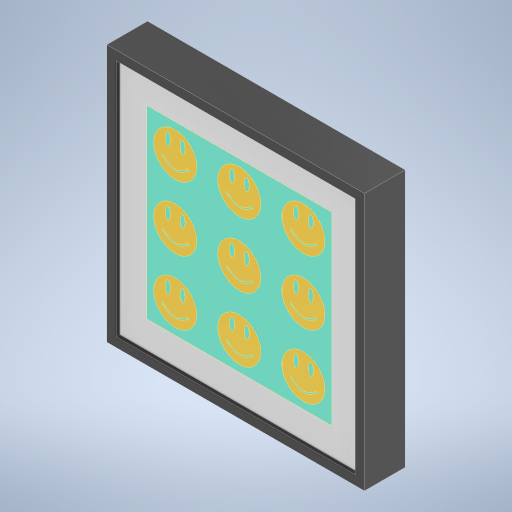
# Autodesk Inventor part: picture-frame-square
Saved by Autodesk Inventor 2023 (Build 270158030, 158C)
## iProperties
Created: 2023-12-24
Part Number: picture-frame-square
Material: Generic
Document SubType Name: Modeling
Designer: Imogen Heard
Density: 1 g/cm^3
Appearance: Glossy - Gold
Author: Imogen Heard
Autodesk Inventor part; units mm, degrees
ref_plane "YZ Plane" through (0, 0, 0) normal (1, 0, 0) x (0, 1, 0)
ref_plane "XZ Plane" through (0, 0, 0) normal (0, 1, 0) x (-1, 0, 0)
ref_plane "XY Plane" through (0, 0, 0) normal (0, 0, 1) x (1, 0, 0)
sketch "Sketch1" plane through (0, 0, 0) normal (0, 0, 1) x (1, 0, 0)
  line L0 (0, 200) -> (200, 200)
  line L1 (200, 200) -> (200, 0)
  line L2 (200, 0) -> (0, 0)
  line L3 (0, 0) -> (0, 200)
  dimension "d0" = 200
  dimension "d1" = 200
  constraints: 8 end point, 2 parallel, 1 coincident, 1 horizontal, 1 perpendicular
  measures "d0" distance between parallel lines of L1 L3
  measures "d1" distance between parallel lines of L2 L0
extrude "Extrusion1" add sketch "Sketch1" along normal blind 0.01
sketch "Sketch2" plane through (0, 0, 0.01) normal (0, 0, 1) x (1, 0, 0)
  line L0 (25, 175) -> (175, 175)
  line L1 (175, 175) -> (175, 25)
  line L2 (175, 25) -> (25, 25)
  line L3 (25, 25) -> (25, 175)
  line L4 (0, 200) -> (0, 0) projected
  line L5 (200, 200) -> (0, 200) projected
  line L6 (200, 0) -> (200, 200) projected
  line L7 (0, 0) -> (200, 0) projected
  dimension "d4" = 25
  dimension "d5" = 25
  dimension "d6" = 25
  dimension "d7" = 25
  constraints: 8 end point, 2 parallel, 1 horizontal, 1 perpendicular
  measures "d4" distance between parallel lines of L4 L3
  measures "d5" distance between parallel lines of L5 L0
  measures "d6" distance between parallel lines of L6 L1
  measures "d7" distance between parallel lines of L7 L2
extrude "Extrusion2" add sketch "Sketch2" along normal blind 0.02 contours L0 L1 L2 L3
sketch "Sketch3" plane through (0, 0, 0.03) normal (0, 0, 1) x (1, 0, 0)
  circle A0 centre (48, 152) radius 17.5
  line L0 (175, 175) -> (25, 175) projected
  line L1 (25, 175) -> (25, 25) projected
  ellipse E0 centre (42, 160) end of major axis (42, 155) minor radius 2
  ellipse E1 centre (54, 160) end of major axis (54, 155) minor radius 2
  line L2 (38.6458, 146.4746) -> (47.8499, 137.8273) construction
  line L3 (47.8499, 137.8273) -> (57.4024, 146.0108) construction
  spline S0 degree 2 poles (38.6458, 146.4746) (47.8499, 137.8273) (57.4024, 146.0108) knots 1 1 1 2 2 2
  ellipse E2 centre (58.0984, 145.8999) end of major axis (58.7934, 145.0887) minor radius 0.5281 (58.0325, 145.2429) -> (57.4024, 146.0108) ccw
  ellipse E3 centre (37.9912, 146.4065) end of major axis (38.6402, 147.2549) minor radius 0.5281 (38.6458, 146.4746) -> (38.0218, 145.6984) ccw
  ellipse E4 centre (89.9912, 146.4065) end of major axis (90.6402, 147.2549) minor radius 0.5281 (90.6458, 146.4746) -> (90.0218, 145.6984) ccw
  ellipse E5 centre (110.0984, 145.8999) end of major axis (110.7934, 145.0887) minor radius 0.5281 (110.0325, 145.2429) -> (109.4024, 146.0108) ccw
  spline S1 degree 2 poles (90.6458, 146.4746) (99.8499, 137.8273) (109.4024, 146.0108) knots 1 1 1 2 2 2
  line L4 (90.6458, 146.4746) -> (99.8499, 137.8273) construction
  line L5 (99.8499, 137.8273) -> (109.4024, 146.0108) construction
  circle A1 centre (100, 152) radius 17.5
  ellipse E6 centre (94, 160) end of major axis (94, 155) minor radius 2
  ellipse E7 centre (106, 160) end of major axis (106, 155) minor radius 2
  ellipse E8 centre (141.9912, 146.4065) end of major axis (142.6402, 147.2549) minor radius 0.5281 (142.6458, 146.4746) -> (142.0218, 145.6984) ccw
  ellipse E9 centre (162.0984, 145.8999) end of major axis (162.7934, 145.0887) minor radius 0.5281 (162.0325, 145.2429) -> (161.4024, 146.0108) ccw
  spline S2 degree 2 poles (142.6458, 146.4746) (151.8499, 137.8273) (161.4024, 146.0108) knots 1 1 1 2 2 2
  line L6 (142.6458, 146.4746) -> (151.8499, 137.8273) construction
  line L7 (151.8499, 137.8273) -> (161.4024, 146.0108) construction
  circle A2 centre (152, 152) radius 17.5
  ellipse E10 centre (146, 160) end of major axis (146, 155) minor radius 2
  ellipse E11 centre (158, 160) end of major axis (158, 155) minor radius 2
  ellipse E12 centre (37.9912, 94.4065) end of major axis (38.6402, 95.2549) minor radius 0.5281 (38.6458, 94.4746) -> (38.0218, 93.6984) ccw
  ellipse E13 centre (58.0984, 93.8999) end of major axis (58.7934, 93.0887) minor radius 0.5281 (58.0325, 93.2429) -> (57.4024, 94.0108) ccw
  spline S3 degree 2 poles (38.6458, 94.4746) (47.8499, 85.8273) (57.4024, 94.0108) knots 1 1 1 2 2 2
  line L8 (38.6458, 94.4746) -> (47.8499, 85.8273) construction
  line L9 (47.8499, 85.8273) -> (57.4024, 94.0108) construction
  circle A3 centre (48, 100) radius 17.5
  ellipse E14 centre (42, 108) end of major axis (42, 103) minor radius 2
  ellipse E15 centre (54, 108) end of major axis (54, 103) minor radius 2
  ellipse E16 centre (89.9912, 94.4065) end of major axis (90.6402, 95.2549) minor radius 0.5281 (90.6458, 94.4746) -> (90.0218, 93.6984) ccw
  ellipse E17 centre (110.0984, 93.8999) end of major axis (110.7934, 93.0887) minor radius 0.5281 (110.0325, 93.2429) -> (109.4024, 94.0108) ccw
  spline S4 degree 2 poles (90.6458, 94.4746) (99.8499, 85.8273) (109.4024, 94.0108) knots 1 1 1 2 2 2
  line L10 (90.6458, 94.4746) -> (99.8499, 85.8273) construction
  line L11 (99.8499, 85.8273) -> (109.4024, 94.0108) construction
  circle A4 centre (100, 100) radius 17.5
  ellipse E18 centre (94, 108) end of major axis (94, 103) minor radius 2
  ellipse E19 centre (106, 108) end of major axis (106, 103) minor radius 2
  ellipse E20 centre (141.9912, 94.4065) end of major axis (142.6402, 95.2549) minor radius 0.5281 (142.6458, 94.4746) -> (142.0218, 93.6984) ccw
  ellipse E21 centre (162.0984, 93.8999) end of major axis (162.7934, 93.0887) minor radius 0.5281 (162.0325, 93.2429) -> (161.4024, 94.0108) ccw
  spline S5 degree 2 poles (142.6458, 94.4746) (151.8499, 85.8273) (161.4024, 94.0108) knots 1 1 1 2 2 2
  line L12 (142.6458, 94.4746) -> (151.8499, 85.8273) construction
  line L13 (151.8499, 85.8273) -> (161.4024, 94.0108) construction
  circle A5 centre (152, 100) radius 17.5
  ellipse E22 centre (146, 108) end of major axis (146, 103) minor radius 2
  ellipse E23 centre (158, 108) end of major axis (158, 103) minor radius 2
  ellipse E24 centre (37.9912, 42.4065) end of major axis (38.6402, 43.2549) minor radius 0.5281 (38.6458, 42.4746) -> (38.0218, 41.6984) ccw
  ellipse E25 centre (58.0984, 41.8999) end of major axis (58.7934, 41.0887) minor radius 0.5281 (58.0325, 41.2429) -> (57.4024, 42.0108) ccw
  spline S6 degree 2 poles (38.6458, 42.4746) (47.8499, 33.8273) (57.4024, 42.0108) knots 1 1 1 2 2 2
  line L14 (38.6458, 42.4746) -> (47.8499, 33.8273) construction
  line L15 (47.8499, 33.8273) -> (57.4024, 42.0108) construction
  circle A6 centre (48, 48) radius 17.5
  ellipse E26 centre (42, 56) end of major axis (42, 51) minor radius 2
  ellipse E27 centre (54, 56) end of major axis (54, 51) minor radius 2
  ellipse E28 centre (89.9912, 42.4065) end of major axis (90.6402, 43.2549) minor radius 0.5281 (90.6458, 42.4746) -> (90.0218, 41.6984) ccw
  ellipse E29 centre (110.0984, 41.8999) end of major axis (110.7934, 41.0887) minor radius 0.5281 (110.0325, 41.2429) -> (109.4024, 42.0108) ccw
  spline S7 degree 2 poles (90.6458, 42.4746) (99.8499, 33.8273) (109.4024, 42.0108) knots 1 1 1 2 2 2
  line L16 (90.6458, 42.4746) -> (99.8499, 33.8273) construction
  line L17 (99.8499, 33.8273) -> (109.4024, 42.0108) construction
  circle A7 centre (100, 48) radius 17.5
  ellipse E30 centre (94, 56) end of major axis (94, 51) minor radius 2
  ellipse E31 centre (106, 56) end of major axis (106, 51) minor radius 2
  ellipse E32 centre (141.9912, 42.4065) end of major axis (142.6402, 43.2549) minor radius 0.5281 (142.6458, 42.4746) -> (142.0218, 41.6984) ccw
  ellipse E33 centre (162.0984, 41.8999) end of major axis (162.7934, 41.0887) minor radius 0.5281 (162.0325, 41.2429) -> (161.4024, 42.0108) ccw
  spline S8 degree 2 poles (142.6458, 42.4746) (151.8499, 33.8273) (161.4024, 42.0108) knots 1 1 1 2 2 2
  line L18 (142.6458, 42.4746) -> (151.8499, 33.8273) construction
  line L19 (151.8499, 33.8273) -> (161.4024, 42.0108) construction
  circle A8 centre (152, 48) radius 17.5
  ellipse E34 centre (146, 56) end of major axis (146, 51) minor radius 2
  ellipse E35 centre (158, 56) end of major axis (158, 51) minor radius 2
  spline S9 degree 5 poles (38.0218, 145.6983) (39.1499, 144.6441) (40.3558, 143.6753) (41.6486, 142.8112) (44.2977, 141.4889) (47.2032, 140.953) (48.6132, 140.9177) (51.5488, 141.3098) (54.2641, 142.5084) (55.601, 143.3166) (56.8543, 144.2346) (58.0325, 145.2429) knots 0 0 0 0 0 0 0.344675 0.344675 0.344675 0.653835 0.653835 0.653835 1 1 1 1 1 1
  spline S10 degree 5 poles (90.0218, 145.6983) (91.1499, 144.6441) (92.3558, 143.6753) (93.6486, 142.8112) (96.2977, 141.4889) (99.2032, 140.953) (100.6132, 140.9177) (103.5488, 141.3098) (106.2641, 142.5084) (107.601, 143.3166) (108.8543, 144.2346) (110.0325, 145.2429) knots 0 0 0 0 0 0 0.344675 0.344675 0.344675 0.653835 0.653835 0.653835 1 1 1 1 1 1
  spline S11 degree 5 poles (142.0218, 145.6983) (143.1499, 144.6441) (144.3558, 143.6753) (145.6486, 142.8112) (148.2977, 141.4889) (151.2032, 140.953) (152.6132, 140.9177) (155.5488, 141.3098) (158.2641, 142.5084) (159.601, 143.3166) (160.8543, 144.2346) (162.0325, 145.2429) knots 0 0 0 0 0 0 0.344675 0.344675 0.344675 0.653835 0.653835 0.653835 1 1 1 1 1 1
  spline S12 degree 5 poles (38.0218, 93.6983) (39.1499, 92.6441) (40.3558, 91.6753) (41.6486, 90.8112) (44.2977, 89.4889) (47.2032, 88.953) (48.6132, 88.9177) (51.5488, 89.3098) (54.2641, 90.5084) (55.601, 91.3166) (56.8543, 92.2346) (58.0325, 93.2429) knots 0 0 0 0 0 0 0.344675 0.344675 0.344675 0.653835 0.653835 0.653835 1 1 1 1 1 1
  spline S13 degree 5 poles (90.0218, 93.6983) (91.1499, 92.6441) (92.3558, 91.6753) (93.6486, 90.8112) (96.2977, 89.4889) (99.2032, 88.953) (100.6132, 88.9177) (103.5488, 89.3098) (106.2641, 90.5084) (107.601, 91.3166) (108.8543, 92.2346) (110.0325, 93.2429) knots 0 0 0 0 0 0 0.344675 0.344675 0.344675 0.653835 0.653835 0.653835 1 1 1 1 1 1
  spline S14 degree 5 poles (142.0218, 93.6983) (143.1499, 92.6441) (144.3558, 91.6753) (145.6486, 90.8112) (148.2977, 89.4889) (151.2032, 88.953) (152.6132, 88.9177) (155.5488, 89.3098) (158.2641, 90.5084) (159.601, 91.3166) (160.8543, 92.2346) (162.0325, 93.2429) knots 0 0 0 0 0 0 0.344675 0.344675 0.344675 0.653835 0.653835 0.653835 1 1 1 1 1 1
  spline S15 degree 5 poles (38.0218, 41.6983) (39.1499, 40.6441) (40.3558, 39.6753) (41.6486, 38.8112) (44.2977, 37.4889) (47.2032, 36.953) (48.6132, 36.9177) (51.5488, 37.3098) (54.2641, 38.5084) (55.601, 39.3166) (56.8543, 40.2346) (58.0325, 41.2429) knots 0 0 0 0 0 0 0.344675 0.344675 0.344675 0.653835 0.653835 0.653835 1 1 1 1 1 1
  spline S16 degree 5 poles (90.0218, 41.6983) (91.1499, 40.6441) (92.3558, 39.6753) (93.6486, 38.8112) (96.2977, 37.4889) (99.2032, 36.953) (100.6132, 36.9177) (103.5488, 37.3098) (106.2641, 38.5084) (107.601, 39.3166) (108.8543, 40.2346) (110.0325, 41.2429) knots 0 0 0 0 0 0 0.344675 0.344675 0.344675 0.653835 0.653835 0.653835 1 1 1 1 1 1
  spline S17 degree 5 poles (142.0218, 41.6983) (143.1499, 40.6441) (144.3558, 39.6753) (145.6486, 38.8112) (148.2977, 37.4889) (151.2032, 36.953) (152.6132, 36.9177) (155.5488, 37.3098) (158.2641, 38.5084) (159.601, 39.3166) (160.8543, 40.2346) (162.0325, 41.2429) knots 0 0 0 0 0 0 0.344675 0.344675 0.344675 0.653835 0.653835 0.653835 1 1 1 1 1 1
  point P0 (0, 0)
  dimension "d10" = 35
  dimension "d11" = 23
  dimension "d12" = 23
  dimension "d13" = 5
  dimension "d14" = 5
  dimension "d15" = 2
  dimension "d16" = 2
  dimension "d17" = 6
  dimension "d18" = 6
  dimension "d19" = 8
  dimension "d22" = 52
  dimension "d25" = 52
  constraints: 27 centre point, 19 vertical, 7 horizontal, 1 equal radius, 1 horizontal alignment, 232 other
  measures "d10" diameter of A0
  measures "d11" distance from line of L0 A0.centre
  measures "d12" distance from line of L1 A0.centre
  measures "d17" horizontal distance of E0.centre A0.centre
  measures "d18" horizontal distance of E1.centre A0.centre
  measures "d19" vertical distance of A0.centre E1.centre
  measures "d22" distance of A0.centre A1.centre
  measures "d25" distance of A0.centre A3.centre
extrude "Extrusion3" add sketch "Sketch3" along normal blind 0.02
sketch "Sketch4" plane through (0, 0, 0) normal (0, 0, -1) x (-1, 0, 0)
  line L0 (-203, 203) -> (3, 203)
  line L1 (3, 203) -> (3, -3)
  line L2 (3, -3) -> (-203, -3)
  line L3 (-203, -3) -> (-203, 203)
  line L4 (0, 200) -> (0, 0) projected
  line L5 (-200, 200) -> (0, 200) projected
  line L6 (-200, 0) -> (-200, 200) projected
  line L7 (0, 0) -> (-200, 0) projected
  dimension "d30" = 3
  dimension "d31" = 3
  dimension "d32" = 3
  dimension "d33" = 3
  constraints: 8 end point, 2 parallel, 1 horizontal, 1 perpendicular
  measures "d30" distance between parallel lines of L4 L1
  measures "d31" distance between parallel lines of L5 L0
  measures "d32" distance between parallel lines of L3 L6
  measures "d33" distance between parallel lines of L2 L7
extrude "Extrusion4" add sketch "Sketch4" along normal blind 2 separate body contours L0 L1 L2 L3 | L4 L7 L6 L5
sketch "Sketch7" plane through (0, 0, -2) normal (0, 0, -1) x (-1, 0, 0)
  line L0 (-203, -3) -> (3, -3) projected
  line L1 (3, -3) -> (3, 203) projected
  line L2 (3, 203) -> (-203, 203) projected
  line L3 (-203, 203) -> (-203, -3) projected
  line L4 (-200, 200) -> (0, 200)
  line L5 (0, 200) -> (0, 0)
  line L6 (0, 0) -> (-200, 0)
  line L7 (-200, 0) -> (-200, 200)
  point P0 (0, 0)
  dimension "d39" = 3
  constraints: 8 end point, 3 other
  measures "d39" distance between parallel lines of L2 L4
extrude "Extrusion6" add sketch "Sketch7" along normal blind 25 bodies 2
sketch "Sketch8" plane through (0, 0, -27) normal (0, 0, -1) x (-1, 0, 0)
  line L0 (3, -3) -> (3, 203) projected
  line L1 (3, 203) -> (-203, 203) projected
  line L2 (-203, 203) -> (-203, -3) projected
  line L3 (-203, -3) -> (3, -3) projected
  line L4 (-200, 200) -> (0, 200) projected
  line L5 (0, 200) -> (0, 0) projected
  line L6 (0, 0) -> (-200, 0) projected
  line L7 (-200, 0) -> (-200, 200) projected
  arc A0 (-92.5, 185) -> (-107.5, 185) centre (-100, 185) ccw
  arc A1 (-152.5, 185) -> (-167.5, 185) centre (-160, 185) ccw
  arc A2 (-32.5, 185) -> (-47.5, 185) centre (-40, 185) ccw
  line L8 (-185, 185) -> (-167.5, 185)
  line L9 (-152.5, 185) -> (-107.5, 185)
  line L10 (-92.5, 185) -> (-47.5, 185)
  line L11 (-32.5, 185) -> (-15, 185)
  circle A3 centre (-100, 100) radius 10
  line L12 (-185, 47.5) -> (-185, 92.5)
  arc A4 (-185, 47.5) -> (-185, 32.5) centre (-185, 40) ccw
  line L13 (-185, 15) -> (-185, 32.5)
  line L14 (-185, 107.5) -> (-185, 152.5)
  arc A5 (-185, 107.5) -> (-185, 92.5) centre (-185, 100) ccw
  arc A6 (-185, 167.5) -> (-185, 152.5) centre (-185, 160) ccw
  line L15 (-185, 167.5) -> (-185, 185)
  line L16 (-47.5, 15) -> (-92.5, 15)
  arc A7 (-47.5, 15) -> (-32.5, 15) centre (-40, 15) ccw
  line L17 (-15, 15) -> (-32.5, 15)
  line L18 (-107.5, 15) -> (-152.5, 15)
  arc A8 (-107.5, 15) -> (-92.5, 15) centre (-100, 15) ccw
  arc A9 (-167.5, 15) -> (-152.5, 15) centre (-160, 15) ccw
  line L19 (-167.5, 15) -> (-185, 15)
  line L20 (-15, 152.5) -> (-15, 107.5)
  arc A10 (-15, 152.5) -> (-15, 167.5) centre (-15, 160) ccw
  line L21 (-15, 185) -> (-15, 167.5)
  line L22 (-15, 92.5) -> (-15, 47.5)
  arc A11 (-15, 92.5) -> (-15, 107.5) centre (-15, 100) ccw
  arc A12 (-15, 32.5) -> (-15, 47.5) centre (-15, 40) ccw
  line L23 (-15, 32.5) -> (-15, 15)
  point P0 (0, 0)
  dimension "d43" = 15
  dimension "d44" = 60
  dimension "d45" = 60
  dimension "d46" = 15
  dimension "d47" = 15
  dimension "d48" = 15
  dimension "d49" = 40
  dimension "d50" = 40
  dimension "d51" = 100
  dimension "d52" = 100
  dimension "d53" = 100
  dimension "d54" = 20
  dimension "d57" = 360
  constraints: 32 end point, 24 point on circle, 13 centre point, 8 horizontal alignment, 2 equal radius, 73 other
  measures "d43" diameter of A0
  measures "d44" distance of A2.centre A0.centre
  measures "d45" distance of A1.centre A0.centre
  measures "d46" distance between parallel lines of L4 L10
  measures "d47" distance from line of L5 L11.end
  measures "d48" distance from line of L7 L8.start
  measures "d49" distance from line of L5 A2.centre
  measures "d50" distance from line of L7 A1.centre
  measures "d51" distance from line of L5 A3.centre
  measures "d52" distance from line of L7 A3.centre
  measures "d53" distance from line of L6 A3.centre
  measures "d54" diameter of A3
extrude "Extrusion7" add sketch "Sketch8" along normal blind 3 contours L3 L2 L1 L0 | L4 L5 L6 L7 bodies 2
sketch "Sketch10" plane through (0, 0, 0.01) normal (0, 0, 1) x (1, 0, 0)
  line L0 (203, -3) -> (-3, -3) projected
  line L1 (203, 203) -> (203, -3) projected
  line L2 (-3, 203) -> (203, 203) projected
  line L3 (-3, -3) -> (-3, 203) projected
  line L4 (204.5, 204.5) -> (204.5, -4.5)
  line L5 (204.5, -4.5) -> (-4.5, -4.5)
  line L6 (-4.5, -4.5) -> (-4.5, 204.5)
  line L7 (-4.5, 204.5) -> (204.5, 204.5)
  line L8 (25, 25) -> (25, 175) projected
  line L9 (25, 175) -> (175, 175) projected
  line L10 (175, 175) -> (175, 25) projected
  line L11 (175, 25) -> (25, 25) projected
  line L12 (0, 0) -> (200, 0) projected
  line L13 (200, 0) -> (200, 200) projected
  line L14 (200, 200) -> (0, 200) projected
  line L15 (0, 200) -> (0, 0) projected
  line L16 (3, 197) -> (197, 197)
  line L17 (197, 197) -> (197, 3)
  line L18 (197, 3) -> (3, 3)
  line L19 (3, 3) -> (3, 197)
  dimension "d61" = 1.5
  dimension "d62" = 3
  constraints: 16 end point, 6 other
  measures "d61" distance between parallel lines of L2 L7
  measures "d62" distance between parallel lines of L16 L14
extrude "Extrusion8" add sketch "Sketch10" along normal blind 3 separate body contours L0 L3 L2 L1 | L4 L5 L6 L7 | L15 L14 L13 L12
sketch "Sketch11" plane through (0, 0, 0.01) normal (0, 0, -1) x (-1, 0, 0)
  line L0 (4.5, 204.5) -> (4.5, -4.5) projected
  line L1 (-204.5, 204.5) -> (4.5, 204.5) projected
  line L2 (-204.5, -4.5) -> (-204.5, 204.5) projected
  line L3 (4.5, -4.5) -> (-204.5, -4.5) projected
  line L4 (-3, 197) -> (-197, 197) projected
  line L5 (-3, 3) -> (-3, 197) projected
  line L6 (-197, 3) -> (-3, 3) projected
  line L7 (-197, 197) -> (-197, 3) projected
  line L8 (3, 203) -> (-203, 203) projected
  line L9 (-203.01, -3.01) -> (-203.01, 203.01)
  line L10 (-203.01, 203.01) -> (3.01, 203.01)
  line L11 (3.01, 203.01) -> (3.01, -3.01)
  line L12 (3.01, -3.01) -> (-203.01, -3.01)
  point P0 (0, 0)
  dimension "d65" = 0.01
  constraints: 8 end point
  measures "d65" distance between parallel lines of L8 L10
extrude "Extrusion9" add sketch "Sketch11" along normal up to surface (30.01 mm away) contours L0 L3 L2 L1 bodies 3
sketch "Sketch6" plane through (0, 0, 0) normal (0, 0, 1) x (1, 0, 0)
  line L0 (203, 203) -> (203, -3) projected
  line L1 (203, -3) -> (-3, -3) projected
  line L2 (203, 203) -> (203, -3) projected
  line L3 (-3, 203) -> (203, 203) projected
  line L4 (-3, -3) -> (-3, 203) projected
  line L5 (25, 25) -> (25, 175) projected
  line L6 (25, 175) -> (175, 175) projected
  line L7 (175, 175) -> (175, 25) projected
  line L8 (175, 25) -> (25, 25) projected
  line L9 (0, 0) -> (200, 0) projected
  line L10 (200, 0) -> (200, 200) projected
  line L11 (200, 200) -> (0, 200) projected
  line L12 (0, 200) -> (0, 0) projected
  line L13 (-1.5, 201.5) -> (201.5, 201.5)
  line L14 (201.5, 201.5) -> (201.5, -1.5)
  line L15 (201.5, -1.5) -> (-1.5, -1.5)
  line L16 (-1.5, -1.5) -> (-1.5, 201.5)
  point P0 (203, -3)
  dimension "d38" = 1.5
  constraints: 8 end point, 3 other
  measures "d38" distance between parallel lines of L4 L16
equation "\"d1\" = d0"
equation "\"d5\" = d4"
equation "\"d6\" = d4"
equation "\"d7\" = d4"
equation "\"d14\" = d13"
equation "\"d16\" = d15"
equation "\"d18\" = d17"
equation "\"d31\" = d30"
equation "\"d32\" = d30"
equation "\"d33\" = d30"
equation "\"d45\" = d44"
equation "\"d47\" = d46"
equation "\"d48\" = d46"
equation "\"d50\" = d49"
